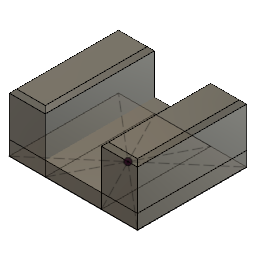
macbookGroundPlug (Autodesk Fusion 360 design; units mm, degrees)
Autodesk Fusion 360 part; units mm, degrees
sketch "Sketch1" plane through (0, 0, 0) normal (0, 1, 0) x (1, 0, 0)
  line L0 (8.8, -7.5) -> (-8.8, -7.5)
  line L1 (-8.8, -7.5) -> (-8.8, 7.5)
  line L2 (-8.8, 7.5) -> (8.8, 7.5)
  line L3 (8.8, 7.5) -> (8.8, -7.5)
  line L4 (8.8, -7.5) -> (-8.8, 7.5) construction
  line L5 (-8.8, -7.5) -> (8.8, 7.5) construction
  line L6 (3.85, -7.5) -> (-3.85, -7.5)
  line L7 (-3.85, -7.5) -> (-3.85, 7.5)
  line L8 (-3.85, 7.5) -> (3.85, 7.5)
  line L9 (3.85, 7.5) -> (3.85, -7.5)
  line L10 (3.85, -7.5) -> (-3.85, 7.5) construction
  line L11 (-3.85, -7.5) -> (3.85, 7.5) construction
  dimension "d1" = 17.6
  dimension "d2" = 15
  dimension "d3" = 7.7
  dimension "d4" = 15
extrude "Extrude1" add sketch "Sketch1" along normal blind 8 contours L0 L2 L3 L9 | L0 L1 L2 L7 makes body 1 at (-8.8, 2.6667, 2.5) makes body 2 at (8.8, 2.6667, -2.5)
extrude "Extrude2" add sketch "Sketch1" along normal blind 2 separate body makes body 3
chamfer "Chamfer1" distance 0.5 angle 45 8 edges at (3.85, 8, 0) (8.8, 8, 0) (6.325, 8, -7.5) (6.325, 8, 7.5) (-8.8, 8, 0) (-3.85, 8, 0) (-6.325, 8, -7.5) (-6.325, 8, 7.5) on bodies 1 2
